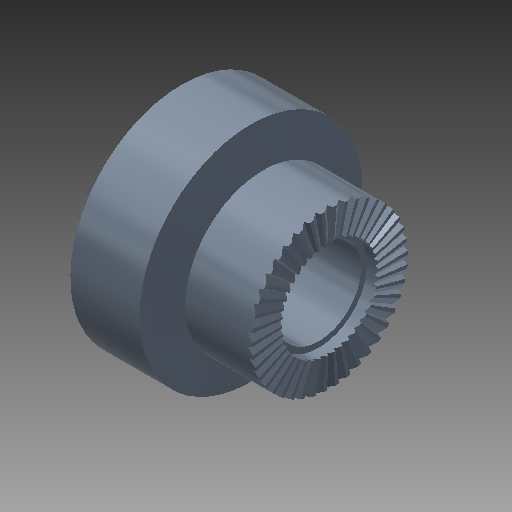
# Autodesk Inventor part: Clutch Prop Mount
Saved by Autodesk Inventor 2017 (Build 210142000, 142)
## iProperties
Created: 2012-08-06
Part Number: Clutch Prop Mount
Material: Stainless Steel, 440C
Document SubType Name: Modeling
Designer: John
Density: 7.75 g/cm^3
Mass: 13.9161 g
Surface Area: 27.6405 cm^2
Volume: 1.79562 cm^3
Appearance: Steel Blue
Author: John
Autodesk Inventor part; units mm, degrees
ref_plane "YZ Plane" through (0, 0, 0) normal (1, 0, 0) x (0, 1, 0)
ref_plane "XZ Plane" through (0, 0, 0) normal (0, 1, 0) x (-1, 0, 0)
ref_plane "XY Plane" through (0, 0, 0) normal (0, 0, 1) x (1, 0, 0)
sketch "Sketch1" plane through (0, 0, 0) normal (1, 0, 0) x (0, 1, 0)
  circle A0 centre (0, 0) radius 12.5095
  dimension "d0" = 25.019
  constraints: 1 centre point, 1 coincident
  measures "d0" diameter of A0
extrude "Extrusion1" add sketch "Sketch1" along normal blind 7.747
sketch "Sketch3" plane through (7.747, 0, 0) normal (1, 0, 0) x (0, 0, -1)
  circle A0 centre (0, 0) radius 12.5095 projected
  circle A1 centre (0, 0) radius 8.763
  dimension "d3" = 17.526
  constraints: 1 centre point, 1 coincident
  measures "d3" diameter of A1
extrude "Extrusion2" add sketch "Sketch3" along normal blind 8.89 contours A1
sketch "Sketch4" plane through (7.747, 0, 0) normal (1, 0, 0) x (0, 0, -1)
  circle A0 centre (0, 0) radius 8.763 projected
  circle A1 centre (0, 0) radius 6.7818
  dimension "d26" = 6.7818
  constraints: 1 centre point
  measures "d26" radius of A1
extrude "Extrusion3" cut sketch "Sketch4" along normal blind 1.397
sketch "Sketch5" plane through (16.637, 0, 0) normal (1, 0, 0) x (0, 0, -1)
  circle A0 centre (0, 0) radius 8.763 projected
hole "Hole1" at (16.637, 0, 0) direction (-1, 0, 0) diameter 9.525 end through all
sketch "Sketch6" plane through (0, 0, 0) normal (-1, 0, 0) x (0, 0, 1)
  circle A0 centre (0, 0) radius 4.7625 projected
hole "Hole2" at (0, 0, 0) direction (1, 0, 0) diameter 23.114 depth 6.8072
sketch "Sketch10" plane through (0, 0, 0) normal (0, 1, 0) x (-1, 0, 0)
  line L0 (-16.637, -4.7625) -> (-16.637, 4.7625) projected
  line L1 (0, 0) -> (-16.637, 0) construction
  line L2 (-16.637, 0.0092) -> (-16.6116, 0)
  line L3 (-16.6116, 0) -> (-16.637, -0.0364)
  dimension "d34" = 75
  dimension "d35" = 0.0254
  constraints: 6 end point, 3 point on line, 1 midpoint
  measures "d34" angle of L3 L2
  measures "d35" distance from line of L0 L2.end
extrude "Extrusion6" cut sketch "Sketch10" against normal through all draft 2
pattern_circular "Circular Pattern1" count 42 over 360 about axis through (-22.4615, 0, 0) along (1, 0, 0) of "Extrusion6"
sketch "Sketch11" plane through (16.637, 0, 0) normal (1, 0, 0) x (0, 0, -1)
  arc A0 (0.5703, -8.7444) -> (0.9745, -8.7086) centre (0, 0) ccw projected
  circle A1 centre (0, 0) radius 5.3975
  dimension "d42" = 10.795
  constraints: 1 centre point, 1 coincident
  measures "d42" diameter of A1
extrude "Extrusion7" cut sketch "Sketch11" against normal blind 1.27
body "Solid1"
